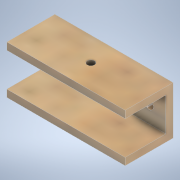
# Autodesk Inventor part: Soporte Motor Izq
Saved by Autodesk Inventor 2021 (Build 250183000, 183)
## iProperties
Created: 2023-01-27
Part Number: Soporte Motor Izq
Material: Madera (arce)
Document SubType Name: Modeling
Designer: Diego.labarca
Density: 0.67 g/cm^3
Appearance: Arce natural - De color oscuro brillante
Author: Diego.labarca
Autodesk Inventor part; units mm, degrees
ref_plane "YZ Plane" through (0, 0, 0) normal (1, 0, 0) x (0, 1, 0)
ref_plane "XZ Plane" through (0, 0, 0) normal (0, 1, 0) x (-1, 0, 0)
ref_plane "XY Plane" through (0, 0, 0) normal (0, 0, 1) x (1, 0, 0)
sketch "Boceto1" plane through (0, 0, 0) normal (0, 0, 1) x (1, 0, 0)
  line L0 (-28.1218, 9.9396) -> (21.1782, 9.9396)
  line L1 (21.1782, 9.9396) -> (21.1782, -10.0604)
  line L2 (21.1782, -10.0604) -> (-28.1218, -10.0604)
  line L3 (-28.1218, -10.0604) -> (-28.1218, 9.9396)
  line L4 (2.6895, 0) -> (0, 0)
  line L5 (0, 0) -> (0, 2.3867)
  dimension "d0" = 20
  dimension "d1" = 49.3
  constraints: 12 end point, 2 horizontal, 2 parallel, 2 perpendicular
  measures "d0" distance of L0.end L1.end
  measures "d1" distance of L0.start L0.end
extrude "Extrusión1" add sketch "Boceto1" along normal blind 3
sketch "Boceto2" plane through (0, 0, 3) normal (0, 0, 1) x (1, 0, 0)
  line L0 (-28.1218, 9.9396) -> (-28.1218, -10.0604) projected
  line L1 (21.1782, -10.0604) -> (21.1782, 9.9396) projected
  line L2 (-28.1218, 9.9396) -> (21.1782, 9.9396)
  line L3 (21.1782, 9.9396) -> (21.1782, 6.9396)
  line L4 (21.1782, 6.9396) -> (-28.1218, 6.9396)
  line L5 (-28.1218, 6.9396) -> (-28.1218, 9.9396)
  line L6 (21.1782, -10.0604) -> (-28.1218, -10.0604)
  line L7 (-28.1218, -10.0604) -> (-28.1218, -7.0604)
  line L8 (-28.1218, -7.0604) -> (21.1782, -7.0604)
  line L9 (21.1782, -7.0604) -> (21.1782, -10.0604)
  point P0 (0, 0)
  dimension "d4" = 3
  dimension "d5" = 3
  constraints: 16 end point, 4 parallel, 2 horizontal, 2 perpendicular, 2 point on line
  measures "d4" distance between parallel lines of L2 L4
  measures "d5" distance between parallel lines of L6 L8
extrude "Extrusión2" add sketch "Boceto2" along normal blind 17 contours L2 L1 L4 L0 | L8 L1 L6 L0
sketch "Boceto3" plane through (0, 0, 3) normal (0, 0, 1) x (1, 0, 0)
  circle A0 centre (-11.8218, 0) radius 1.75
  line L0 (-28.1218, 6.9396) -> (-28.1218, -7.0604) projected
  circle A1 centre (14.1782, -0.0604) radius 1.75
  line L1 (21.1782, -7.0604) -> (21.1782, 6.9396) projected
  point P0 (0, 0)
  dimension "d8" = 3.5
  dimension "d10" = 3.5
  dimension "d16" = 7
  dimension "d17" = 33
  constraints: 2 centre point
  measures "d8" diameter of A0
  measures "d10" diameter of A1
  measures "d16" distance from line of L1 A1.centre
  measures "d17" distance from line of A0.centre L1
extrude "Extrusión3" cut sketch "Boceto3" against normal through all
sketch "Boceto4" plane through (-28.1218, 9.9396, 0) normal (0, 1, 0) x (1, 0, 0)
  circle A0 centre (25, -10) radius 1.5
  line L0 (49.3, -20) -> (0, -20) projected
  line L1 (49.3, 0) -> (49.3, -20) projected
  point P0 (28.1218, 0)
  dimension "d18" = 3
  dimension "d19" = 10
  dimension "d20" = 24.3
  constraints: 1 centre point
  measures "d18" diameter of A0
  measures "d19" distance from line of A0.centre L0
  measures "d20" distance from line of L1 A0.centre
extrude "Extrusión4" cut sketch "Boceto4" against normal up to surface (3 mm away)
equation "\"d10\" = d8"
